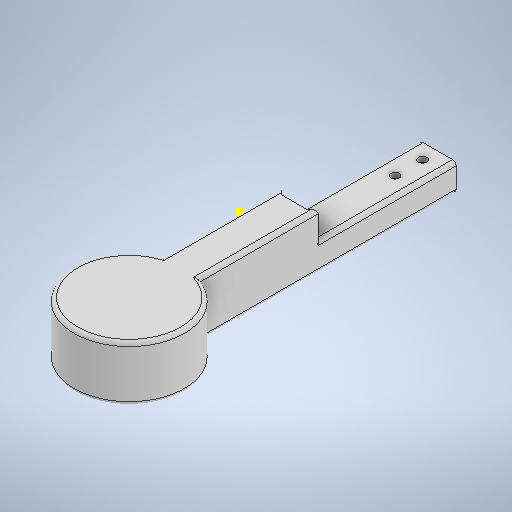
# Autodesk Inventor part: shotHolder
Saved by Autodesk Inventor 2025 (Build 290162000, 162)
## iProperties
Created: 2024-05-22
Part Number: shotHolder
Material: Generic
Document SubType Name: Modeling
Designer: 48791
Density: 1 g/cm^3
Appearance: Default
Author: 48791
Autodesk Inventor part; units mm, degrees
ref_plane "YZ Plane" through (0, 0, 0) normal (1, 0, 0) x (0, 1, 0)
ref_plane "XZ Plane" through (0, 0, 0) normal (0, 1, 0) x (-1, 0, 0)
ref_plane "XY Plane" through (0, 0, 0) normal (0, 0, 1) x (1, 0, 0)
sketch "Sketch1" plane through (0, 0, 0) normal (0, 1, 0) x (-1, 0, 0)
  line L0 (0, 0) -> (-20, 0)
  line L1 (-20, 0) -> (-20, -100)
  line L2 (-20, -100) -> (0, -100)
  line L3 (0, -100) -> (0, 0)
  dimension "d0" = 20
  dimension "d1" = 100
  constraints: 8 end point, 2 parallel, 1 horizontal, 1 perpendicular
  measures "d0" distance of L2.end L1.end
  measures "d1" distance of L0.end L1.end
extrude "Extrusion1" add sketch "Sketch1" along normal blind 15
sketch "Sketch2" plane through (0, 15, 0) normal (0, 1, 0) x (1, 0, 0)
  line L0 (20, 0) -> (20, 100) projected
  line L1 (0, 100) -> (0, 0) projected
  line L2 (20, 0) -> (0, 0)
  line L3 (0, 0) -> (0, 19.5)
  line L4 (0, 19.5) -> (20, 19.5)
  line L5 (20, 19.5) -> (20, 0)
  dimension "d4" = 19.5
  constraints: 8 end point, 2 parallel, 1 horizontal, 1 perpendicular, 1 point on line
  measures "d4" distance between parallel lines of L2 L4
extrude "Extrusion2" add sketch "Sketch2" along normal blind 15
sketch "Sketch3" plane through (0, 15, 0) normal (0, 1, 0) x (1, 0, 0)
  line L0 (20, 19.5) -> (0, 19.5) projected
  line L1 (0, 19.5) -> (0, 22.5)
  line L2 (0, 100) -> (0, 0) projected
  line L3 (0, 22.5) -> (3.0005, 19.5)
  line L4 (3.0005, 19.5) -> (0, 19.5)
  line L5 (20, 19.5) -> (20, 22.5)
  line L6 (20, 0) -> (20, 100) projected
  line L7 (20, 22.5) -> (16.9995, 19.5)
  line L8 (16.9995, 19.5) -> (20, 19.5)
  dimension "d7" = 3
  dimension "d8" = 4.243
  dimension "d9" = 3
  dimension "d10" = 4.243
  constraints: 12 end point, 3 point on line, 2 perpendicular
  measures "d7" distance of L0.end L1.end
  measures "d8" distance of L1.end L3.end
  measures "d9" distance of L0.start L5.end
  measures "d10" distance of L5.end L7.end
extrude "Extrusion3" add sketch "Sketch3" along normal blind 15
sketch "Sketch4" plane through (0, 0, 0) normal (0, 0, 1) x (1, 0, 0)
  point P0 (0, 0)
sketch "Sketch5" plane through (0, 0, 0) normal (0, 0, 1) x (1, 0, 0)
  line L0 (0, 0) -> (20, 0) projected
  line L1 (20, 30) -> (16.9995, 30) projected
  line L2 (0, 0) -> (20, 0)
  line L3 (20, 0) -> (20, 30)
  line L4 (20, 30) -> (0, 30)
  line L5 (0, 30) -> (0, 0)
  constraints: 8 end point, 2 parallel, 1 horizontal, 1 perpendicular
extrude "Extrusion4" add sketch "Sketch5" along normal blind 80
sketch "Sketch6" plane through (0, 0, 80) normal (0, 0, 1) x (1, 0, 0)
  line L0 (19, 3) -> (1, 3)
  line L1 (1, 3) -> (1, 12)
  line L2 (1, 12) -> (19, 12)
  line L3 (19, 12) -> (19, 3)
  line L4 (0, 30) -> (0, 0) projected
  line L5 (0, 0) -> (20, 0) projected
  dimension "d15" = 18
  dimension "d16" = 9
  dimension "d17" = 1
  dimension "d18" = 3
  constraints: 8 end point, 2 parallel, 1 horizontal, 1 perpendicular
  measures "d15" distance of L1.end L2.end
  measures "d16" distance between parallel lines of L2 L0
  measures "d17" distance between parallel lines of L4 L1
  measures "d18" distance between parallel lines of L5 L0
extrude "Extrusion5" cut sketch "Sketch6" against normal blind 160
sketch "Sketch7" plane through (0, 0, 0) normal (0, -1, 0) x (1, 0, 0)
  circle A0 centre (10, -89.5) radius 2.25
  circle A1 centre (10, -74.5) radius 2.25
  line L0 (20, -100) -> (0, -100) projected
  line L1 (0, -100) -> (0, 80) projected
  point P0 (0, 0)
  point P1 (10, -100)
  dimension "d21" = 4.5
  dimension "d22" = 4.5
  dimension "d23" = 10.5
  dimension "d24" = 10.5
  dimension "d25" = 10
  dimension "d26" = 10
  constraints: 2 centre point, 1 midpoint
  measures "d21" diameter of A0
  measures "d22" diameter of A1
  measures "d23" distance of point (10, -100) A0.centre
  measures "d25" distance from line of L1 A0.centre
  measures "d26" distance from line of L1 A1.centre
extrude "Extrusion6" cut sketch "Sketch7" against normal blind 160
sketch "Sketch8" plane through (0, 0, -80) normal (0, 0, 1) x (1, 0, 0)
  line L0 (19, 3) -> (1, 3) projected
  line L1 (1, 12) -> (19, 12) projected
  line L2 (19, 3) -> (1, 3)
  line L3 (1, 3) -> (1, 12)
  line L4 (1, 12) -> (19, 12)
  line L5 (19, 12) -> (19, 3)
  point P0 (0, 0)
  constraints: 8 end point, 2 parallel, 1 horizontal, 1 perpendicular
extrude "Extrusion7" add sketch "Sketch8" along normal blind 170
sketch "Sketch9" plane through (0, 30, 0) normal (0, 1, 0) x (1, 0, 0)
  point P0 (0, 0)
sketch "Sketch10" plane through (0, 0, 90) normal (0, 0, 1) x (1, 0, 0)
  line L0 (19, 3) -> (1, 3) projected
  line L1 (1, 12) -> (19, 12) projected
  line L2 (1, 3) -> (19, 3)
  line L3 (19, 3) -> (19, 12)
  line L4 (19, 12) -> (1, 12)
  line L5 (1, 12) -> (1, 3)
  point P0 (0, 0)
  constraints: 8 end point, 2 parallel, 1 horizontal, 1 perpendicular
extrude "Extrusion8" cut sketch "Sketch10" against normal blind 185
sketch "Sketch11" plane through (0, 15, 0) normal (0, 1, 0) x (1, 0, 0)
  line L0 (0, 100) -> (0, -80) projected
  line L1 (20, -80) -> (20, 100) projected
  line L2 (0, 100) -> (20, 100)
  line L3 (20, 100) -> (20, 97.7472)
  line L4 (20, 97.7472) -> (0, 97.7472)
  line L5 (0, 97.7472) -> (0, 100)
  point P0 (0, 0)
  point P1 (0, 97.7472)
  constraints: 8 end point, 2 parallel, 1 horizontal, 1 perpendicular, 1 point on line
extrude "Extrusion9" cut sketch "Sketch11" against normal blind 185
sketch "Sketch12" plane through (0, 30, 0) normal (0, 1, 0) x (1, 0, 0)
  circle A0 centre (10, -70.4515) radius 30
  point P0 (0, 0)
  dimension "d35" = 60
  constraints: 1 centre point
  measures "d35" diameter of A0
extrude "Extrusion10" add sketch "Sketch12" along normal mid plane 60
sketch "Sketch13" plane through (10, 60, 70.4515) normal (0, 1, 0) x (1, 0, 0)
  circle A0 centre (0, 0) radius 30
  point P0 (-10, 70.4515)
  constraints: 1 centre point
extrude "Extrusion11" cut sketch "Sketch13" against normal blind 30
sketch "Sketch14" plane through (0, 30, 0) normal (0, 1, 0) x (1, 0, 0)
  point P0 (0, 0)
sketch "Sketch15" plane through (0, 0, 0) normal (0, -1, 0) x (1, 0, 0)
  arc A0 (1, 41.8333) -> (19, 41.8333) centre (10, 70.4515) ccw projected
  circle A1 centre (4.9424, 40.8809) radius 2.5
  circle A2 centre (15.0576, 40.8809) radius 2.5
  point P0 (0, 0)
  dimension "d40" = 5
  dimension "d41" = 5
  constraints: 2 centre point, 2 point on circle
  measures "d40" diameter of A1
  measures "d41" diameter of A2
extrude "Extrusion12" cut sketch "Sketch15" against normal blind 13
sketch "Sketch16" plane through (0, 0, 0) normal (0, -1, 0) x (1, 0, 0)
  circle A0 centre (10, -89.5) radius 2.25 projected
  circle A1 centre (10, -89.5) radius 3.5
  circle A2 centre (10, -74.5) radius 2.25 projected
  circle A3 centre (10, -74.5) radius 3.5
  point P0 (0, 0)
  dimension "d44" = 7
  dimension "d45" = 7
  constraints: 2 centre point, 2 coincident
  measures "d44" diameter of A1
  measures "d45" diameter of A3
extrude "Extrusion13" cut sketch "Sketch16" against normal blind 6
fillet "Fillet1" radius 2 8 edges at (20, 30, 9.8336) (20, 15, -60.1236) (0, 15, -60.1236) (0, 30, 9.8336) (0, 0, -27.79) (20, 0, -27.79) (10, 30, 100.4515) (10, 0, 100.4515)
sketch "Sketch17" plane through (0, 0, 0) normal (0, -1, 0) x (1, 0, 0)
  circle A0 centre (10, 22.1222) radius 2.4
  line L0 (2, -97.7472) -> (2, 43.6187) projected
  point P0 (0, 0)
  dimension "d49" = 4.8
  dimension "d50" = 8
  constraints: 1 centre point
  measures "d49" diameter of A0
  measures "d50" distance from line of L0 A0.centre
extrude "Extrusion14" cut sketch "Sketch17" against normal blind 6
body "Solid1"
